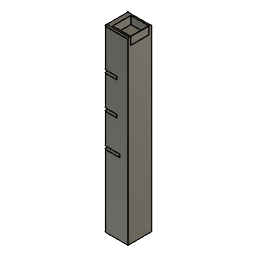
sensor-rod (Autodesk Fusion 360 design; units mm, degrees)
part number: 2026-07-21-11-04-03-204
Autodesk Fusion 360 part; units mm, degrees
note: some values were not read from the file. Set by a fixed rule: which sketch regions a step uses.
sketch "Sketch1" plane through (0, 0, 0) normal (0, 0, 1) x (1, 0, 0)
  line L0 (9.925, 9.925) -> (-9.925, 9.925)
  line L1 (-9.925, 9.925) -> (-9.925, -9.925)
  line L2 (-9.925, -9.925) -> (9.925, -9.925)
  line L3 (9.925, -9.925) -> (9.925, 9.925)
  line L4 (9.925, 9.925) -> (-9.925, -9.925) construction
  line L5 (-9.925, 9.925) -> (9.925, -9.925) construction
  dimension "d1" = 19.85
  dimension "d2" = 19.85
  constraint horizontal L0
  constraint perpendicular L0 L1
  constraint parallel L0 L2
  constraint parallel L1 L3
  constraint coincident L4 origin
  constraint coincident L5 origin
  measures "d1" distance of L1.end L2.end
  measures "d2" distance of L0.end L1.end
extrude "Extrude1" add sketch "Sketch1" along normal blind 150
sketch "Sketch2" plane through (0, -9.925, 0) normal (0, -1, 0) x (1, 0, 0)
  line L0 (-9.925, 0) -> (9.925, 0)
  line L1 (9.925, 0) -> (9.925, 150)
  line L2 (9.925, 150) -> (-9.925, 150)
  line L3 (-9.925, 150) -> (-9.925, 0)
  line L4 (-9.925, 62.54) -> (2.925, 62.54)
  line L5 (2.925, 62.54) -> (2.925, 60)
  line L6 (2.925, 60) -> (-9.925, 60)
  line L7 (-9.925, 60) -> (-9.925, 62.54)
  line L8 (-9.925, 90.08) -> (0.535, 90.08)
  line L9 (0.535, 90.08) -> (0.535, 87.54)
  line L10 (0.535, 87.54) -> (-9.925, 87.54)
  line L11 (-9.925, 87.54) -> (-9.925, 90.08)
  line L12 (-9.925, 117.62) -> (0.535, 117.62)
  line L13 (0.535, 117.62) -> (0.535, 115.08)
  line L14 (0.535, 115.08) -> (-9.925, 115.08)
  line L15 (-9.925, 115.08) -> (-9.925, 117.62)
  dimension "d5" = 12.85
  dimension "d6" = 2.54
  dimension "d7" = 60
  dimension "d8" = 10.46
  dimension "d9" = 2.54
  dimension "d10" = 25
  dimension "d11" = 10.46
  dimension "d12" = 2.54
  dimension "d13" = 25
  constraint horizontal L4
  constraint vertical L5
  constraint horizontal L6
  constraint vertical L7
  constraint coincident L3 L4.start
  constraint horizontal L8
  constraint vertical L9
  constraint horizontal L10
  constraint vertical L11
  constraint coincident L3 L8.start
  constraint horizontal L12
  constraint vertical L13
  constraint horizontal L14
  constraint vertical L15
  constraint coincident L3 L12.start
  measures "d5" distance of L4.start L4.end
  measures "d6" distance of L4.start L6.end
  measures "d7" distance of L0 L6
  measures "d8" distance of L8.start L8.end
  measures "d9" distance of L8.start L10.end
  measures "d10" distance of L4 L10
  measures "d11" distance of L12.start L12.end
  measures "d12" distance of L12.start L14.end
  measures "d13" distance of L8 L14
extrude "Extrude2" cut sketch "Sketch2" against normal blind 30 contours L3 L4 L5 L6 L7 | L3 L8 L9 L10 L11 | L3 L12 L13 L14 L15
fillet "Fillet1" radius 1 8 edges at (-9.925, -9.925, 133.81) (-9.925, -9.925, 102.58) (-9.925, -9.925, 75.04) (-9.925, -9.925, 30) (-9.925, 9.925, 133.81) (-9.925, 9.925, 102.58) (-9.925, 9.925, 75.04) (-9.925, 9.925, 30)
fillet "Fillet2" radius 1 5 edges at (0.5, 9.925, 150) (-9.6321, 9.6321, 150) (-9.925, 0, 150) (-9.6321, -9.6321, 150) (0.5, -9.925, 150)
sketch "Sketch3" plane through (-9.925, 0, 0) normal (-1, 0, 0) x (0, -1, 0)
  line L0 (8.925, 149) -> (-8.925, 149)
  line L1 (-8.925, 149) -> (-8.925, 117.62)
  line L2 (-8.925, 117.62) -> (8.925, 117.62)
  line L3 (8.925, 117.62) -> (8.925, 149)
  line L4 (5.075, 129.62) -> (-4.925, 129.62)
  line L5 (-4.925, 129.62) -> (-4.925, 123.62)
  line L6 (-4.925, 123.62) -> (5.075, 123.62)
  line L7 (5.075, 123.62) -> (5.075, 129.62)
  line L8 (5.075, 129.62) -> (-4.925, 123.62) construction
  line L9 (-4.925, 129.62) -> (5.075, 123.62) construction
  line L10 (-4.9698, 54) -> (5.0302, 54)
  line L11 (5.0302, 54) -> (5.0302, 48)
  line L12 (5.0302, 48) -> (-4.9698, 48)
  line L13 (-4.9698, 48) -> (-4.9698, 54)
  line L14 (-4.9698, 54) -> (5.0302, 48) construction
  line L15 (5.0302, 54) -> (-4.9698, 48) construction
  line L16 (8.925, 60) -> (-8.925, 60)
  point P0 (0.075, 126.62)
  point P1 (0.0302, 51)
  dimension "d20" = 10
  dimension "d21" = 6
  dimension "d22" = 3.85
  dimension "d23" = 6
  dimension "d24" = 6
  dimension "d25" = 10
  dimension "d26" = 6
  constraint horizontal L4
  constraint perpendicular L4 L5
  constraint parallel L4 L6
  constraint parallel L5 L7
  constraint coincident L8 P0
  constraint coincident L9 P0
  constraint horizontal L10
  constraint perpendicular L10 L11
  constraint parallel L10 L12
  constraint parallel L11 L13
  constraint coincident L14 P1
  constraint coincident L15 P1
  constraint collinear origin P0 P1
  measures "d20" distance of L5.end L6.end
  measures "d21" distance of L4.end L5.end
  measures "d22" distance of L3 L7
  measures "d23" distance of L2 L6
  measures "d24" distance of L10.end L11.end
  measures "d25" distance of L10.start L10.end
  measures "d26" distance of L10 L16
extrude "Extrude3" cut sketch "Sketch3" against normal blind 5 contours L4 L5 L6 L7 | L10 L11 L12 L13
sketch "Sketch4" plane through (0, 0, 150) normal (0, 0, 1) x (-1, 0, 0)
  line L0 (8.925, 8.925) -> (-9.925, 8.925)
  line L1 (-9.925, 8.925) -> (-9.925, -8.925)
  line L2 (-9.925, -8.925) -> (8.925, -8.925)
  line L3 (8.925, -8.925) -> (8.925, 8.925)
  line L4 (-9.775, -7.625) -> (5.225, -7.625)
  line L5 (5.225, -7.625) -> (5.225, 7.575)
  line L6 (5.225, 7.575) -> (-9.775, 7.575)
  line L7 (-9.775, 7.575) -> (-9.775, -7.625)
  line L8 (-9.775, -7.625) -> (5.225, 7.575) construction
  line L9 (5.225, -7.625) -> (-9.775, 7.575) construction
  point P0 (-2.275, -0.025)
  dimension "d29" = 15
  dimension "d30" = 15.2
  dimension "d31" = 1.3
  dimension "d32" = 3.7
  constraint horizontal L4
  constraint perpendicular L4 L5
  constraint parallel L4 L6
  constraint parallel L5 L7
  constraint coincident L8 P0
  constraint coincident L9 P0
  measures "d29" distance of L5.end L6.end
  measures "d30" distance of L4.end L5.end
  measures "d31" distance of L2 L4
  measures "d32" distance of L3 L5
extrude "Extrude4" cut sketch "Sketch4" against normal blind 6.6 contours L4 L5 L6 L7
sketch "Sketch7" plane through (-9.925, 0, 0) normal (-1, 0, 0) x (0, -1, 0)
  line L0 (-4.925, 129.62) -> (5.075, 129.62)
  line L1 (5.075, 129.62) -> (5.075, 123.62)
  line L2 (5.075, 123.62) -> (-4.925, 123.62)
  line L3 (-4.925, 123.62) -> (-4.925, 129.62)
  line L4 (8.925, 149) -> (-8.925, 149)
  line L5 (-8.925, 149) -> (-8.925, 117.62)
  line L6 (-8.925, 117.62) -> (8.925, 117.62)
  line L7 (8.925, 117.62) -> (8.925, 149)
  line L8 (5.075, 143.62) -> (-4.925, 143.62)
  line L9 (-4.925, 143.62) -> (-4.925, 137.62)
  line L10 (-4.925, 137.62) -> (5.075, 137.62)
  line L11 (5.075, 137.62) -> (5.075, 143.62)
  line L12 (5.075, 143.62) -> (-4.925, 137.62) construction
  line L13 (-4.925, 143.62) -> (5.075, 137.62) construction
  line L14 (5.0197, 34) -> (-4.9803, 34)
  line L15 (-4.9803, 34) -> (-4.9803, 40)
  line L16 (-4.9803, 40) -> (5.0197, 40)
  line L17 (5.0197, 40) -> (5.0197, 34)
  line L18 (5.0197, 34) -> (-4.9803, 40) construction
  line L19 (-4.9803, 34) -> (5.0197, 40) construction
  line L20 (5.0302, 48) -> (-4.9698, 48)
  point P0 (0.075, 140.62)
  point P1 (0.0197, 37)
  dimension "d45" = 8
  dimension "d46" = 3.85
  dimension "d47" = 6
  dimension "d48" = 10
  dimension "d49" = 6
  dimension "d50" = 8
  constraint horizontal L8
  constraint perpendicular L8 L9
  constraint parallel L8 L10
  constraint parallel L9 L11
  constraint coincident L12 P0
  constraint coincident L13 P0
  constraint collinear L3 L9
  constraint horizontal L14
  constraint perpendicular L14 L15
  constraint parallel L14 L16
  constraint parallel L15 L17
  constraint coincident L18 P1
  constraint coincident L19 P1
  constraint collinear origin P0 P1
  measures "d45" distance of L0 L10
  measures "d46" distance of L7 L11
  measures "d47" distance of L8 L10
  measures "d48" distance of L15.end L16.end
  measures "d49" distance of L14.end L15.end
  measures "d50" distance of L16 L20
extrude "Extrude6" cut sketch "Sketch7" against normal blind 4 contours L8 L9 L10 L11 | L14 L15 L16 L17
